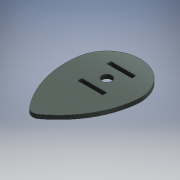
# Autodesk Inventor part: leva00
Saved by Autodesk Inventor 2016 (Build 200138000, 138)
## iProperties
Created: 2016-09-20
Part Number: leva00
Material: Madera (abedul)
Document SubType Name: Modeling
Designer: i95sa
Density: 0.55 g/cm^3
Appearance: Gris plomo - Pulido
Author: i95sa
Autodesk Inventor part; units mm, degrees
ref_plane "YZ Plane" through (0, 0, 0) normal (1, 0, 0) x (0, 1, 0)
ref_plane "XZ Plane" through (0, 0, 0) normal (0, 1, 0) x (-1, 0, 0)
ref_plane "XY Plane" through (0, 0, 0) normal (0, 0, 1) x (1, 0, 0)
sketch "Boceto1" plane through (0, 0, 0) normal (0, 0, 1) x (1, 0, 0)
  arc A0 (4.2118, 33.34) -> (-4.2118, -33.34) centre (0, 0) ccw
  arc A1 (-6.4817, -51.3077) -> (-8.4256, -66.6954) centre (-7.4536, -59.0015) ccw
  line L0 (-8.707, -68.9229) -> (-16.4008, -67.951)
  line L1 (-33.2878, 4.6065) -> (-46.1109, 6.2264)
  line L2 (-46.1109, 6.2264) -> (-16.4008, -67.951)
  line L3 (-16.4008, -67.951) -> (-27.9345, -39.1549)
  arc A2 (-33.2878, 4.6065) -> (-27.9345, -39.1549) centre (51.8943, -7.1813) ccw
  arc A3 (-27.9345, -39.1549) -> (-13.4999, -63.8577) centre (62.2103, -3.0495) ccw
  line L4 (0.324, 2.5646) -> (4.2118, 33.34)
  line L5 (-0.324, -2.5646) -> (-8.707, -68.9229)
  arc A4 (-4.2118, -33.34) -> (4.2118, 33.34) centre (0, 0) ccw
  arc A5 (-8.4256, -66.6954) -> (-6.4817, -51.3077) centre (-7.4536, -59.0015) ccw
  line L6 (-8.707, -68.9229) -> (-1.0131, -69.8949)
  line L7 (33.3876, -3.8166) -> (46.2107, -5.4365)
  line L8 (46.2107, -5.4365) -> (-1.0131, -69.8949)
  line L9 (-1.0131, -69.8949) -> (17.3194, -44.8717)
  arc A6 (17.3194, -44.8717) -> (33.3876, -3.8166) centre (-52.0499, 5.9499) ccw
  arc A7 (-2.805, -65.2088) -> (17.3194, -44.8717) centre (-61.0142, 12.5174) ccw
  dimension "d0" = 67.21
  dimension "d6" = 15.51
  dimension "d7" = 7.755
  dimension "d8" = 12.925
  dimension "d9" = 31.02
  constraints: 20 end point, 20 point on circle, 8 centre point, 6 symmetric about line, 5 point on line, 4 tangent, 1 collinear, 4 other
  measures "d0" diameter of A0
  measures "d6" diameter of A1
  measures "d7" distance of L0.start L0.end
  measures "d8" distance of L1.start L1.end
  measures "d9" distance of L0.end L3.end
extrude "Extrusión2" add sketch "Boceto1" along normal blind 4 contours A4 A0 | A0 L5 A1 A3 A2 | A6 A7 A5 L5 A4 | L5 A1 | A5 L5
sketch "Boceto2" plane through (0, 0, 4) normal (0, 0, 1) x (1, 0, 0)
  line L0 (0, 0) -> (0, 12.5)
  line L1 (0, 12.5) -> (-12.5, 12.5)
  line L2 (-12.5, 12.5) -> (-12.5, 16.7)
  line L3 (-12.5, 16.7) -> (12.5, 16.7)
  line L4 (12.5, 16.7) -> (12.5, 12.5)
  line L5 (12.5, 12.5) -> (0, 12.5)
  line L6 (0, 0) -> (12.5, 0)
  line L7 (0, 0) -> (0, -12.5)
  line L8 (0, -12.5) -> (-12.5, -12.5)
  line L9 (-12.5, -12.5) -> (-12.5, -16.7)
  line L10 (-12.5, -16.7) -> (12.5, -16.7)
  line L11 (12.5, -16.7) -> (12.5, -12.5)
  line L12 (12.5, -12.5) -> (0, -12.5)
  circle A0 centre (0, 0) radius 5
  dimension "d24" = 12.5
  dimension "d25" = 12.5
  dimension "d26" = 4.2
  dimension "d27" = 25
  dimension "d28" = 10
  constraints: 26 end point, 5 perpendicular, 5 symmetric about line, 3 point on line, 1 centre point, 1 coincident, 1 parallel, 1 vertical
  measures "d24" distance of L0.start L0.end
  measures "d25" distance of L0.end L1.end
  measures "d26" distance of L1.end L2.end
  measures "d27" distance of L2.end L3.end
  measures "d28" diameter of A0
extrude "Extrusión3" cut sketch "Boceto2" against normal blind 4
